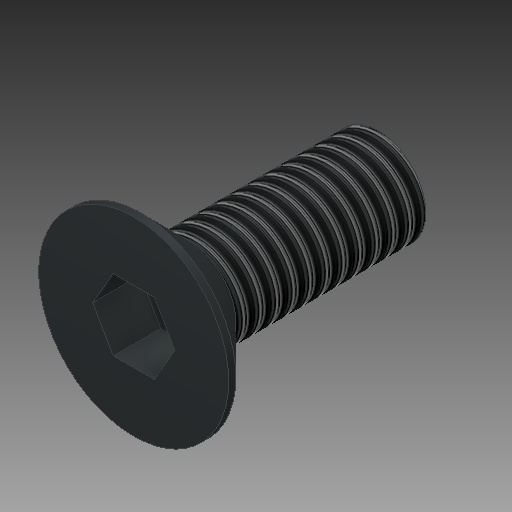
# Autodesk Inventor part: M4皿ネジ　8
Saved by Autodesk Inventor 2017.3 (Build 213256000, 256)
## iProperties
Part Number: M4皿ネジ　8
Material: 鉄 灰色
Document SubType Name: Modeling
Designer: 原知也
Density: 7.15 g/cm^3
Appearance: 鉄 灰色
Mass: 1.13446 g
Surface Area: 2.45002 cm^2
Volume: 0.158665 cm^3
Author: 原知也
Autodesk Inventor part; units mm, degrees
ref_plane "YZ Plane" through (0, 0, 0) normal (1, 0, 0) x (0, 1, 0)
ref_plane "XZ Plane" through (0, 0, 0) normal (0, 1, 0) x (-1, 0, 0)
ref_plane "XY Plane" through (0, 0, 0) normal (0, 0, 1) x (1, 0, 0)
sketch "スケッチ1" plane through (0, 0, 0) normal (0, 0, 1) x (1, 0, 0)
  circle A0 centre (0, 0) radius 2
  dimension "d0" = 4
  constraints: 1 centre point, 1 coincident
  measures "d0" diameter of A0
extrude "押し出し1" add sketch "スケッチ1" along normal blind 8
sketch "スケッチ2" plane through (0, 0, 8) normal (0, 0, 1) x (1, 0, 0)
  circle A0 centre (0, 0) radius 4
  dimension "d3" = 8
  constraints: 1 centre point, 1 coincident
  measures "d3" diameter of A0
extrude "押し出し2" add sketch "スケッチ2" along normal blind 2.3
chamfer "面取り1" distance 2 angle 45 1 edges at (-4, 0, 8)
sketch "スケッチ3" plane through (0, 0, 10.3) normal (0, 0, 1) x (1, 0, 0)
  line L0 (1.7321, 0) -> (0.866, -1.5)
  line L1 (0.866, -1.5) -> (-0.866, -1.5)
  line L2 (-0.866, -1.5) -> (-1.7321, 0)
  line L3 (-1.7321, 0) -> (-0.866, 1.5)
  line L4 (-0.866, 1.5) -> (0.866, 1.5)
  line L5 (0.866, 1.5) -> (1.7321, 0)
  point P0 (0, 0)
  point P1 (0, 0)
  dimension "d9" = 3
  constraints: 12 end point, 1 coincident, 13 other
  measures "d9" distance between parallel lines of L2 L5
extrude "押し出し3" cut sketch "スケッチ3" against normal blind 2
thread "ねじ1" size "M4x0.7" class "6g" standard "ANSI Metric M Profile" full length
